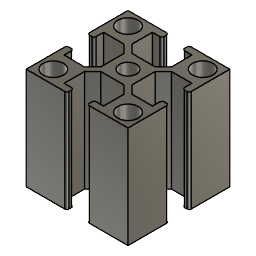
LDO_1515_Cube (Autodesk Fusion 360 design; units mm, degrees)
Autodesk Fusion 360 part; units mm, degrees
sketch "Cross Section" plane through (0, 0, 0) normal (0, 0, 1) x (1, 0, 0)
  line L0 (-7.5, -7.5) -> (7.5, -7.5)
  line L1 (7.5, -7.5) -> (7.5, 7.5)
  line L2 (7.5, 7.5) -> (-7.5, 7.5)
  line L3 (-7.5, -1.8) -> (-7.5, -7.5)
  line L4 (-7.5, -7.5) -> (7.5, 7.5) construction
  line L5 (7.5, -7.5) -> (-7.5, 7.5) construction
  line L6 (-7.2, 1.5) -> (-6.8, 1.5)
  line L7 (-6.5, 1.8) -> (-6.5, 2.9)
  line L8 (-6.5, 2.9) -> (-3.5, 2.9)
  line L9 (-3.5, 2.9) -> (-2.3, 1.7)
  line L10 (-2.3, 1.7) -> (-2.3, -1.7)
  line L11 (-2.3, -1.7) -> (-3.5, -2.9)
  line L12 (-3.5, -2.9) -> (-6.5, -2.9)
  line L13 (-6.5, -2.9) -> (-6.5, -1.8)
  line L14 (-6.8, -1.5) -> (-7.2, -1.5)
  line L15 (-2.3, 0) -> (-7.5, 0) construction
  circle A0 centre (0, 0) radius 1.25
  circle A1 centre (-5.5, 5.5) radius 1.5
  line L16 (-7.5, -7.5) -> (-7.5, -1.5)
  line L17 (-7.5, 1.8) -> (-7.5, 7.5)
  arc A2 (-7.5, 1.8) -> (-7.2, 1.5) centre (-7.2, 1.8) ccw
  arc A3 (-6.8, 1.5) -> (-6.5, 1.8) centre (-6.8, 1.8) ccw
  arc A4 (-6.5, -1.8) -> (-6.8, -1.5) centre (-6.8, -1.8) ccw
  arc A5 (-7.2, -1.5) -> (-7.5, -1.8) centre (-7.2, -1.8) ccw
  arc A6 (-1.8, -7.5) -> (-1.5, -7.2) centre (-1.8, -7.2) ccw
  line L18 (-1.5, -7.2) -> (-1.5, -6.8)
  line L19 (2.9, -6.5) -> (1.8, -6.5)
  arc A7 (1.8, -6.5) -> (1.5, -6.8) centre (1.8, -6.8) ccw
  line L20 (1.5, -6.8) -> (1.5, -7.2)
  arc A8 (1.5, -7.2) -> (1.8, -7.5) centre (1.8, -7.2) ccw
  line L21 (2.9, -3.5) -> (2.9, -6.5)
  line L22 (1.7, -2.3) -> (2.9, -3.5)
  line L23 (-1.7, -2.3) -> (1.7, -2.3)
  line L24 (-2.9, -3.5) -> (-1.7, -2.3)
  line L25 (-2.9, -6.5) -> (-2.9, -3.5)
  line L26 (-1.8, -6.5) -> (-2.9, -6.5)
  arc A9 (-1.5, -6.8) -> (-1.8, -6.5) centre (-1.8, -6.8) ccw
  line L27 (7.5, -7.5) -> (1.5, -7.5)
  line L28 (-1.8, -7.5) -> (-7.5, -7.5)
  circle A10 centre (-5.5, -5.5) radius 1.5
  arc A11 (7.5, -1.8) -> (7.2, -1.5) centre (7.2, -1.8) ccw
  line L29 (7.2, -1.5) -> (6.8, -1.5)
  line L30 (6.5, 2.9) -> (6.5, 1.8)
  arc A12 (6.5, 1.8) -> (6.8, 1.5) centre (6.8, 1.8) ccw
  line L31 (6.8, 1.5) -> (7.2, 1.5)
  arc A13 (7.2, 1.5) -> (7.5, 1.8) centre (7.2, 1.8) ccw
  line L32 (3.5, 2.9) -> (6.5, 2.9)
  line L33 (2.3, 1.7) -> (3.5, 2.9)
  line L34 (2.3, -1.7) -> (2.3, 1.7)
  line L35 (3.5, -2.9) -> (2.3, -1.7)
  line L36 (6.5, -2.9) -> (3.5, -2.9)
  line L37 (6.5, -1.8) -> (6.5, -2.9)
  arc A14 (6.8, -1.5) -> (6.5, -1.8) centre (6.8, -1.8) ccw
  line L38 (7.5, 7.5) -> (7.5, 1.5)
  line L39 (7.5, -1.8) -> (7.5, -7.5)
  circle A15 centre (5.5, -5.5) radius 1.5
  arc A16 (1.8, 7.5) -> (1.5, 7.2) centre (1.8, 7.2) ccw
  line L40 (1.5, 7.2) -> (1.5, 6.8)
  line L41 (-2.9, 6.5) -> (-1.8, 6.5)
  arc A17 (-1.8, 6.5) -> (-1.5, 6.8) centre (-1.8, 6.8) ccw
  line L42 (-1.5, 6.8) -> (-1.5, 7.2)
  arc A18 (-1.5, 7.2) -> (-1.8, 7.5) centre (-1.8, 7.2) ccw
  line L43 (-2.9, 3.5) -> (-2.9, 6.5)
  line L44 (-1.7, 2.3) -> (-2.9, 3.5)
  line L45 (1.7, 2.3) -> (-1.7, 2.3)
  line L46 (2.9, 3.5) -> (1.7, 2.3)
  line L47 (2.9, 6.5) -> (2.9, 3.5)
  line L48 (1.8, 6.5) -> (2.9, 6.5)
  arc A19 (1.5, 6.8) -> (1.8, 6.5) centre (1.8, 6.8) ccw
  line L49 (-7.5, 7.5) -> (-1.5, 7.5)
  line L50 (1.8, 7.5) -> (7.5, 7.5)
  circle A20 centre (5.5, 5.5) radius 1.5
  dimension "d2" = 3
  dimension "d3" = 5.2
  dimension "d4" = 5.8
  dimension "d5" = 7.5
  dimension "d6" = 1
  dimension "d7" = 135
  dimension "d8" = 3
  dimension "d9" = 7.5
  dimension "d10" = 2.5
  dimension "d11" = 3
  dimension "d12" = 2
  dimension "d47" = 15
  dimension "d50" = 0.3
  dimension "d52" = 360
  constraint horizontal L0
  constraint perpendicular L0 L1
  constraint parallel L0 L2
  constraint parallel L1 L3
  constraint coincident L4 A0.centre
  constraint coincident L5 A0.centre
  constraint coincident A0.centre origin
  constraint perpendicular L3 L6
  constraint perpendicular L6 L7
  constraint perpendicular L7 L8
  constraint perpendicular L6 L10
  constraint perpendicular L10 L12
  constraint perpendicular L12 L13
  constraint coincident L3 L16.end
  constraint perpendicular L3 L14
  constraint equal L9 L11
  constraint midpoint L10 L15.start
  constraint coincident L3 L15.end
  constraint perpendicular L3 L15
  constraint symmetric L6 L14 L15
  constraint symmetric L8 L12 L15
  constraint coincident L5 A1.centre
  constraint tangent L6 A2
  constraint tangent L17 A2
  constraint tangent L7 A3
  constraint tangent L6 A3
  constraint equal A2 A3
  constraint tangent L14 A4
  constraint tangent L13 A4
  constraint equal A2 A4
  constraint coincident L16.end L14
  constraint coincident L2.end L3
  constraint tangent L14 A5
  constraint tangent L3 A5
  constraint equal A2 A5
  constraint vertical L17
  constraint equal L0 L1
  constraint collinear L7 L13
  measures "d2" distance of L6 L14
  measures "d3" distance of L3 L10
  measures "d4" distance of L8 L12
  measures "d5" distance of L2 L15
  measures "d6" distance of L3 L7
  measures "d7" angle of L9 L10
  measures "d8" distance of L7 L8.end
  measures "d9" distance of L3 A0.centre
  measures "d10" diameter of A0
  measures "d11" diameter of A1
  measures "d12" distance of L3 A1.centre
  measures "d47" distance of L0.start L2.end
  measures "d50" radius of A2
extrude "Extrude1" add sketch "Cross Section" along normal mid plane 15 contours L0 L1 L2 L3 L6 L7 L8 L9 L10 L11 L12 L13 L14 L16 L17 A2 A3 A4 A5 A6 L18 L19 A7 L20 A8 L21 L22 L23 L24 L25 L26 A9 L27 L28 A11 L29 L30 A12 L31 A13 L32 L33 L34 L35 L36 L37 A14 L38 L39 A16 L40 L41 A17 L42 A18 L43 L44 L45 L46 L47 L48 A19 L49 L50
equation "Extrusion_Length = 15 mm"
equation "d20 = Extrusion_Length"
